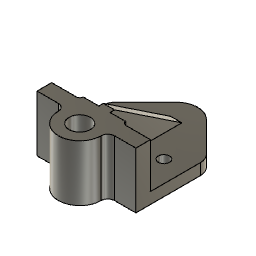
object A3 (Autodesk Fusion 360 design; units mm, degrees)
Autodesk Fusion 360 part; units mm, degrees
note: some values were not read from the file. Set by a fixed rule: which sketch regions a step uses.
sketch "base sketch" plane through (0, 0, 0) normal (0, 0, 1) x (1, 0, 0)
  line L0 (-44, 15.5) -> (44, 15.5)
  line L1 (44, 15.5) -> (44, -15.5)
  line L2 (44, -15.5) -> (-44, -15.5)
  line L3 (-44, -15.5) -> (-44, 15.5)
  line L4 (-44, 15.5) -> (-44, 34.3701)
  line L5 (44, 15.5) -> (44, 34.3701)
  line L6 (-26.8701, 51.5) -> (26.8701, 51.5)
  line L7 (0, -15.5) -> (0, 51.5)
  line L8 (-19, -12.5) -> (-19, -15.5)
  line L9 (19, -12.5) -> (19, -15.5)
  line L10 (-19, -12.5) -> (19, -12.5)
  line L11 (-5, -12.5) -> (-5, -8.5)
  line L12 (5, -12.5) -> (5, -8.5)
  line L13 (-5, -8.5) -> (5, -8.5)
  circle A0 centre (-25, 15.5) radius 5
  circle A1 centre (25, 15.5) radius 5
  circle A2 centre (0, 51.5) radius 19
  line L14 (0, 51.5) -> (13.435, 64.935)
  line L15 (0, 51.5) -> (19, 51.5) construction
  line L16 (0, 51.5) -> (-13.435, 64.935)
  line L17 (-13.435, 64.935) -> (-44, 34.3701)
  line L18 (13.435, 64.935) -> (44, 34.3701)
  line L19 (-44, -15.5) -> (44, -15.5)
  line L20 (44, -15.5) -> (44, -28.5)
  line L21 (-44, -28.5) -> (-44, -15.5)
  circle A3 centre (0, -34.5) radius 9.5
  circle A4 centre (0, -34.5) radius 19
  line L22 (44, -28.5) -> (18.0278, -28.5)
  line L23 (-18.0278, -28.5) -> (-44, -28.5)
  line L24 (-44, -28.5) -> (-18.0278, -28.5)
  line L25 (18.0278, -28.5) -> (44, -28.5)
  dimension "d2" = 31
  dimension "d10" = 38
  dimension "d11" = 25
  dimension "d12" = 4
  dimension "d13" = 4
  dimension "d14" = 39
  dimension "d15" = 10
  dimension "d16" = 10
  dimension "d17" = 10
  dimension "d18" = 50
  dimension "d19" = 19
  dimension "d20" = 38
  dimension "d21" = 45
  dimension "d27" = 13
  dimension "d30" = 19
  dimension "d31" = 38
  constraint horizontal L0
  constraint perpendicular L0 L1
  constraint parallel L0 L2
  constraint parallel L1 L3
  constraint vertical L4
  constraint perpendicular L0 L5
  constraint midpoint L2 L7.start
  constraint coincident L2 L8.end
  constraint perpendicular L2 L8
  constraint coincident L2 L9.end
  constraint perpendicular L2 L9
  constraint coincident L10 L11.start
  constraint perpendicular L10 L11
  constraint coincident L10 L12.start
  constraint perpendicular L10 L12
  constraint coincident L0 A0.centre
  constraint coincident L0 A1.centre
  constraint coincident L7.end A2.centre
  constraint horizontal L15
  constraint tangent A2 L17
  constraint tangent A2 L18
  constraint horizontal L19
  constraint vertical L20
  constraint horizontal L22
  constraint vertical L21
  constraint horizontal L24
  constraint concentric A3 A4
  constraint coincident A4 L23.start
  constraint collinear L22 L23
  constraint collinear L24 L25
  constraint coincident A4 L22.end
  constraint coincident L17 L6.start
  constraint coincident L6 L7.end
  constraint coincident L18 L6.end
  measures "d2" distance of L0.end L1.end
  measures "d10" distance of L8 L9
  measures "d11" distance of L3 L8
  measures "d12" distance of L11.start L11.end
  measures "d13" distance of L12.start L12.end
  measures "d14" distance of L3 L11
  measures "d15" distance of L11 L12
  measures "d16" diameter of A0
  measures "d17" diameter of A1
  measures "d18" distance of A0.centre A1.centre
  measures "d19" distance of L5 A1.centre
  measures "d20" diameter of A2
  measures "d21" angle of L14 L15
  measures "d27" distance of L2.end L21.start
  measures "d30" diameter of A3
  measures "d31" diameter of A4
extrude "Extrude1" add sketch "base sketch" along normal blind 10 contours L0 L5 L6 L7 A1 A2 L18 | L0 L1 L2 L7 L9 L10 L12 L13 A1 L19 | L0 L2 L3 L7 L8 L10 L11 L13 A0 L19 | L0 L4 L6 L7 A0 A2 L17 | L6 A2 L18 | L6 L7 A2 | L6 L7 A2 | L6 A2 L14 | A2 L14 L16 | L6 A2 L16 | L6 A2 L17 makes body 1
extrude "Extrude2" add sketch "base sketch" along normal blind 50 contours L2 L19 L20 A4 L22 L25 | L2 L7 L9 L10 L19 | L7 L10 L12 L13 | L7 L10 L11 L13 | L2 L19 L21 A4 L23 L24 | L2 L7 L8 L10 L19 | A4 bodies 1
fillet "Fillet1" radius 13 1 edges at (44, 34.3701, 5) on bodies 1
fillet "Fillet2" radius 13 1 edges at (-44, 34.3701, 5) on bodies 1
fillet "Fillet3" radius 3 1 edges at (-19, -15.5, 30) on bodies 1
fillet "Fillet4" radius 3 1 edges at (19, -15.5, 30) on bodies 1
fillet "Fillet5" radius 6 1 edges at (18.0278, -28.5, 25) on bodies 1
fillet "Fillet6" radius 6 1 edges at (-18.0278, -28.5, 25) on bodies 1
sketch "slope sketch" plane through (0, 0, 0) normal (1, 0, 0) x (0, 1, 0)
  line L0 (-8.5, 0) -> (51.5, 0)
  line L1 (-8.5, 0) -> (-8.5, 10)
  line L2 (-8.5, 10) -> (51.5, 10)
  line L3 (51.5, 10) -> (51.5, 0)
  line L4 (-8.5, 10) -> (-8.5, 50)
  line L5 (-8.5, 50) -> (51.5, 10)
  dimension "d48" = 60
  dimension "d49" = 40
  constraint horizontal L0
  constraint perpendicular L0 L1
  constraint perpendicular L1 L2
  constraint perpendicular L2 L4
  measures "d48" distance of L1.end L2.end
  measures "d49" distance of L1.end L4.end
extrude "Extrude3" add sketch "slope sketch" along normal mid plane 10 contours L2 L4 L5 bodies 1
copy_body "Body->Comp1" bodies 1 removing the originals makes body 2 in component "object A3"
component "object A3" placed x (1, 0, 0) y (0, 1, 0) z (0, 0, 1) at (0, 0, 0)
named bodies: "object A3"
